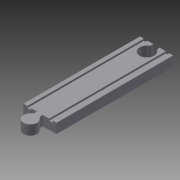
# Autodesk Inventor part: Straight Track
Saved by Autodesk Inventor 2015 (Build 190159000, 159)
## iProperties
Created: 2018-03-28
Part Number: Straight Track
Material: Generic
Document SubType Name: Modeling
Designer: Administrator
Density: 1 g/cm^3
Appearance: Default
Author: Administrator
Autodesk Inventor part; units mm, degrees
ref_plane "YZ Plane" through (0, 0, 0) normal (1, 0, 0) x (0, 1, 0)
ref_plane "XZ Plane" through (0, 0, 0) normal (0, 1, 0) x (-1, 0, 0)
ref_plane "XY Plane" through (0, 0, 0) normal (0, 0, 1) x (1, 0, 0)
sketch "Sketch1" plane through (0, 0, 0) normal (0, 1, 0) x (-1, 0, 0)
  line L0 (64.2981, 132.08) -> (64.2981, -172.72)
  line L1 (64.2981, -172.72) -> (29.3731, -172.72)
  line L2 (29.3731, -172.72) -> (29.3731, -164.4885)
  line L3 (64.2981, 132.08) -> (28.7381, 132.08)
  line L4 (28.7381, 132.08) -> (28.7381, 141.4156)
  line L5 (13.4981, 141.4156) -> (13.4981, 132.08)
  line L6 (13.4981, 132.08) -> (-22.0619, 132.08)
  line L7 (-22.0619, 132.08) -> (-22.0619, -172.72)
  line L8 (-22.0619, -172.72) -> (12.8631, -172.72)
  line L9 (12.8631, -172.72) -> (12.8631, -164.4885)
  arc A0 (28.7381, 141.4156) -> (13.4981, 141.4156) centre (21.1181, 157.48) ccw
  arc A1 (29.3731, -164.4885) -> (12.8631, -164.4885) centre (21.1181, -147.32) ccw
  point P0 (0, 0)
  dimension "d0" = 86.36
  dimension "d1" = 19.05
  dimension "d2" = 17.78
  dimension "d3" = 25.4
  dimension "d4" = 25.4
  dimension "d5" = 304.8
  dimension "d6" = 304.8
  dimension "d7" = 0
  dimension "d8" = 34.925
  dimension "d9" = 51.435
  dimension "d10" = 43.18
  dimension "d13" = 43.18
  dimension "d16" = 15.24
  dimension "d17" = 7.62
  constraints: 20 end point, 6 perpendicular, 4 point on circle, 2 centre point, 2 vertical, 1 horizontal
  measures "d0" distance between parallel lines of L7 L0
  measures "d1" radius of A1
  measures "d2" radius of A0
  measures "d3" distance from line of A0.centre L3
  measures "d4" distance from line of L1 A1.centre
  measures "d5" distance between parallel lines of L8 L6
  measures "d6" distance between parallel lines of L1 L3
  measures "d7" distance between parallel lines of L8 L1
  measures "d8" distance of L0.end L1.end
  measures "d9" distance between parallel lines of L0 L9
  measures "d10" distance from line of L0 A1.centre
  measures "d13" distance from line of L0 A0.centre
  measures "d16" distance between parallel lines of L5 L4
  measures "d17" distance from line of L4 A0.centre
extrude "Extrusion1" add sketch "Sketch1" along normal blind 25.4
sketch "Sketch2" plane through (0, 25.4, 0) normal (0, 1, 0) x (1, 0, 0)
  line L0 (-64.2981, -132.08) -> (-28.7381, -132.08) projected
  line L1 (-13.4981, -132.08) -> (22.0619, -132.08) projected
  line L2 (-29.3731, 172.72) -> (-64.2981, 172.72) projected
  line L3 (22.0619, 172.72) -> (-12.8631, 172.72) projected
  line L4 (-64.2981, 172.72) -> (-64.2981, -132.08) projected
  line L5 (22.0619, -132.08) -> (22.0619, 172.72) projected
  line L6 (-54.1381, -132.08) -> (-54.1381, 172.72)
  line L7 (-64.2981, 172.72) -> (-29.3731, 172.72) projected
  line L8 (-45.2481, 172.72) -> (-45.2481, -132.08)
  line L9 (-54.1381, -132.08) -> (-45.2481, -132.08)
  line L10 (-54.1381, 172.72) -> (-45.2481, 172.72)
  line L11 (3.0119, -132.08) -> (3.0119, 172.72)
  line L12 (11.9019, 172.72) -> (11.9019, -132.08)
  line L13 (3.0119, -132.08) -> (11.9019, -132.08)
  line L14 (3.0119, 172.72) -> (11.9019, 172.72)
  point P0 (0, 0)
  dimension "d21" = 10.16
  dimension "d22" = 19.05
  dimension "d23" = 67.31
  dimension "d24" = 76.2
  constraints: 16 end point, 8 point on line, 4 collinear, 4 perpendicular
  measures "d21" distance between parallel lines of L6 L4
  measures "d22" distance between parallel lines of L4 L8
  measures "d23" distance between parallel lines of L11 L4
  measures "d24" distance between parallel lines of L12 L4
extrude "Extrusion2" cut sketch "Sketch2" against normal blind 4.7625 contours L6 L2 L8 L0 | L11 L3 L12 L1
fillet "Fillet1" radius 4.826 4 edges at (-28.7381, 12.7, 141.4156) (-13.4981, 12.7, 141.4156) (-29.3731, 12.7, -164.4885) (-12.8631, 12.7, -164.4885)
body "Solid1"
